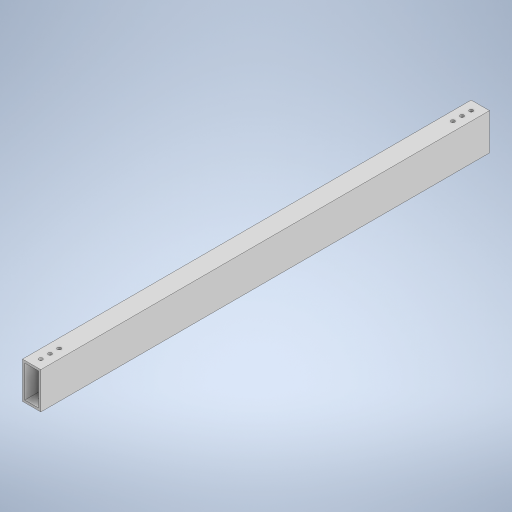
# Autodesk Inventor part: (middle_alum)swerve
Saved by Autodesk Inventor 2024 (Build 280153000, 153)
## iProperties
Created: 2023-10-02
Part Number: (middle_alum)swerve
Material: Generic
Document SubType Name: Modeling
Designer: s137416
Density: 1 g/cm^3
Appearance: Default
Author: s137416
Autodesk Inventor part; units mm, degrees
ref_plane "YZ Plane" through (0, 0, 0) normal (1, 0, 0) x (0, 1, 0)
ref_plane "XZ Plane" through (0, 0, 0) normal (0, 1, 0) x (-1, 0, 0)
ref_plane "XY Plane" through (0, 0, 0) normal (0, 0, 1) x (1, 0, 0)
sketch "Sketch1" plane through (0, 0, 0) normal (0, 1, 0) x (-1, 0, 0)
  line L0 (6.2846, 226.5828) -> (-19.1154, 226.5828)
  line L1 (-19.1154, 226.5828) -> (-19.1154, -395.7172)
  line L2 (-19.1154, -395.7172) -> (6.2846, -395.7172)
  line L3 (6.2846, -395.7172) -> (6.2846, 226.5828)
  circle A0 centre (-6.4154, 213.8828) radius 2.5019
  circle A1 centre (-6.4154, 201.1828) radius 2.5019
  circle A2 centre (-6.4154, 188.4828) radius 2.5019
  circle A3 centre (-6.4154, -383.0172) radius 2.5019
  circle A4 centre (-6.4154, -370.3172) radius 2.5019
  circle A5 centre (-6.4154, -357.6172) radius 2.5019
  point P0 (0, 0)
  point P1 (-6.4154, 226.5828)
  dimension "d0" = 25.4
  dimension "d1" = 622.3
  dimension "d14" = 5.0038
  dimension "d15" = 5.0038
  dimension "d16" = 5.0038
  dimension "d17" = 5.0038
  dimension "d18" = 5.0038
  dimension "d19" = 5.0038
  dimension "d20" = 12.7
  dimension "d21" = 12.7
  dimension "d22" = 12.7
  dimension "d23" = 12.7
  dimension "d24" = 12.7
  dimension "d25" = 12.7
  constraints: 8 end point, 6 centre point, 2 parallel, 1 horizontal, 1 midpoint, 1 perpendicular
  measures "d0" distance of L2.end L1.end
  measures "d1" distance of L2.end L0.start
  measures "d14" diameter of A0
  measures "d15" diameter of A1
  measures "d16" diameter of A2
  measures "d17" diameter of A3
  measures "d18" diameter of A4
  measures "d19" diameter of A5
  measures "d20" distance from line of L2 A3.centre
  measures "d21" distance of A3.centre A4.centre
  measures "d22" distance of A4.centre A5.centre
  measures "d23" distance from line of L0 A0.centre
  measures "d24" distance of A0.centre A1.centre
  measures "d25" distance of A1.centre A2.centre
extrude "Extrusion1" add sketch "Sketch1" along normal blind 50.8
shell "Shell1" thickness 3.175 removed faces 8 at (2.1821, 33.8667, 226.5828) at (8.7885, 16.9333, 213.0905) at (8.7885, 16.9333, 200.3905) at (3.9216, 33.8667, 188.2815) at (10.6487, 33.8667, -395.7172) at (3.9216, 33.8667, -383.2185) at (8.1485, 33.8667, -368.5128) at (3.9216, 33.8667, -357.8185)
body "Solid1"
